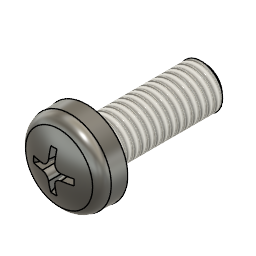
Assembly (Autodesk Fusion 360 archive; units mm, degrees)
design "Tornillo de cabeza plana redondeada ISO 7045 - M3 x 8 - H Acero 4.6 Normal"
description: Tornillo de cabeza plana redondeada ISO 7045 - M3 x 8 - H
part number: ISO 7045 - M3 x 8 - H Acero 4.6 Normal
Autodesk Fusion 360 part; units mm, degrees
sketch "Sketch1" plane through (0, 0, 0) normal (0, 1, 0) x (1, 0, 0)
  line L0 (-1.5, 1) -> (-1.5, 8)
  line L1 (-1.5, 8) -> (0, 8)
  line L2 (0, 8) -> (0, -2.4)
  line L3 (-1.3647, 0) -> (-2.8, 0)
  arc A0 (-2.7449, -1.5792) -> (0, -2.4) centre (0, 2.6) ccw
  line L4 (-1.5, 1) -> (-1.3647, 0.7098)
  line L5 (-1.3647, 0.7098) -> (-1.3647, 0)
  line L6 (-2.8, 0) -> (-2.7449, -1.5792)
  dimension "d9" = 3
  dimension "d66" = 5.6
  dimension "d75" = 2.7294
  dimension "d77" = 1
  dimension "d78" = 155
  dimension "d103" = 2
  dimension "d111" = 2.4
  dimension "d112" = 8
  constraint perpendicular L0 L1
  constraint collinear origin L2.end L1.end
  constraint perpendicular L0 L3
  constraint coincident origin L3
  constraint vertical L0
  constraint vertical L2
  constraint coincident L2 A0.centre
  constraint perpendicular L3 L5
  constraint coincident L3.start L5.end
  measures "d77" distance of L3 L0.start
  measures "d78" angle of L0 L4
  measures "d103" angle of L2 L6
  measures "d111" distance of L2.end L3
  measures "d112" distance of origin L1
revolve "Revolve1" add sketch "Sketch1" angle 360 about axis through (0, 0, -8) along (0, 0, 1) makes body 1
ref_plane "WorkPlane1" through (0, 0, 2.4) normal (0, 0, 1) x (1, 0, 0)
sketch "Sketch2" plane through (0, 0, 2.4) normal (0, 0, 1) x (1, 0, 0)
  line L0 (-0.215, 0.215) -> (-1.5, 0.215)
  line L1 (-0.215, -0.215) -> (-1.5, -0.215)
  line L2 (-1.5, 0.215) -> (-1.5, -0.215)
  line L3 (-0.215, -0.215) -> (-0.215, -1.5)
  line L4 (-0.215, -1.5) -> (0.215, -1.5)
  line L5 (0.215, -0.215) -> (0.215, -1.5)
  line L6 (0.215, -0.215) -> (1.5, -0.215)
  line L7 (1.5, -0.215) -> (1.5, 0.215)
  line L8 (0.215, 0.215) -> (1.5, 0.215)
  line L9 (0.215, 0.215) -> (0.215, 1.5)
  line L10 (0.215, 1.5) -> (-0.215, 1.5)
  line L11 (-0.215, 0.215) -> (-0.215, 1.5)
  dimension "d105" = 0.43
  dimension "d107" = 360
  dimension "d108" = 3
  constraint perpendicular L1 L2
  constraint vertical L0.start L1.start
  constraint horizontal L1
  constraint coincident L8.start L9.start
  measures "d105" distance of L0 L1
  measures "d108" distance of L2 L7
extrude "Extrude1" add sketch "Sketch2" against normal blind 1.8 draft -4 separate body makes body 2
draft "Draft1" angle -30 neutral plane through (0, 0, 2.4) pull (0, 0, 1) 4 faces at (-1.458, -0.0297, 1.8) (0.0297, -1.458, 1.8) (1.458, -0.0297, 1.8) (0.0297, 1.458, 1.8) on bodies 2
fillet "Fillet3" radius 0.43 4 edges at (0.1521, 0.1521, 1.5) (-0.1521, 0.1521, 1.5) (0.1521, -0.1521, 1.5) (-0.1521, -0.1521, 1.5) on bodies 2
combine "Combine1" operation cut target body 1 tool bodies 2
fillet "Fillet4" radius 0.9 1 edges at (-2.5591, 0.9926, 1.5792) on bodies 1
thread "Thread1" "ISO Metric profile 3.0 M3x0.5 M3x0.5 6g" major diameter 2.927 minor diameter 2.3555 pitch 0.5 angle 60 resizes the face on face at (-1.4925, 0.1494, -3.3333) on bodies 1
fillet "Fillet5" radius 0.3 1 edges at (-1.2723, 0.4935, 0) on bodies 1
sketch "Sketch5" plane through (0, 0, 0) normal (0, 1, 0) x (1, 0, 0)
  line L0 (-1.53, 8) -> (-1.53, 7.6933)
  line L1 (-1.53, 7.6933) -> (-1.1933, 8)
  line L2 (0, 8) -> (0, -2.4)
  line L3 (-1.53, 8) -> (0, 8)
  dimension "d114" = 0.3067
  dimension "d115" = 1.53
  dimension "d116" = 0.3367
  constraint coincident L2.start L3.end
  constraint perpendicular L2 L3
  constraint coincident L1.end L3
  constraint perpendicular L0 L3
  measures "d114" distance of L0.end L3
  measures "d115" distance of L0 L2.start
  measures "d116" distance of L0 L1.end
revolve "Revolve2" cut sketch "Sketch5" angle 360 about axis through (0, 0, -8) along (0, 0, 1) bodies 1
equation "d9 = adsk_nomdia"
equation "adsk_nomlen = 8.00 mm"
equation "adsk_headh = 2.40 mm"
equation "adsk_headdia = 5.60 mm"
equation "adsk_nomdia = 3.00 mm"
equation "adsk_phildia = 3.00 mm"
equation "d31 = -adsk_phildepth"
equation "adsk_philwidth = 0.43 mm"
equation "adsk_phildepth = 1.80 mm"
equation "d66 = adsk_headdia"
equation "d71 = adsk_headh"
equation "adsk_thrlen = 7.00 mm"
equation "d75 = adsk_shnkdia"
equation "adsk_shnkdia = 2.72937 mm"
equation "d77 = adsk_nomlen - adsk_thrlen"
equation "adsk_endpointdia = 2.38655 mm"
equation "adsk_startlen = 0.306725 mm"
equation "adsk_ovalrad = 5.00 mm"
equation "adsk_headtoprad = adsk_nomdia * 0.3"
equation "adsk_midfillet = adsk_nomdia * 0.1"
equation "d98 = adsk_midfillet"
equation "adsk_headang = 2.00 deg"
equation "d102 = adsk_headtoprad"
equation "d103 = adsk_headang"
equation "d105 = adsk_philwidth"
equation "d108 = adsk_phildia"
equation "d110 = adsk_philwidth"
equation "d111 = adsk_headh"
equation "d112 = adsk_nomlen"
equation "d113 = ( adsk_nomlen + adsk_headh ) - ( adsk_ovalrad )"
equation "d114 = adsk_startlen"
equation "d115 = adsk_nomdia * 0.51"
equation "d116 = ( adsk_nomdia * 0.51 ) - ( adsk_endpointdia / 2 )"

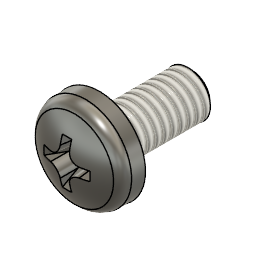
design "Tornillo de cabeza plana redondeada ISO 7045 - M4 x 8 - H Acero 4.6 Normal"
description: Tornillo de cabeza plana redondeada ISO 7045 - M4 x 8 - H
part number: ISO 7045 - M4 x 8 - H Acero 4.6 Normal
Autodesk Fusion 360 part; units mm, degrees
sketch "Sketch1" plane through (0, 0, 0) normal (0, 1, 0) x (1, 0, 0)
  line L0 (-2, 1.4) -> (-2, 8)
  line L1 (-2, 8) -> (0, 8)
  line L2 (0, 8) -> (0, -3.1)
  line L3 (-1.8106, 0) -> (-4, 0)
  arc A0 (-3.9381, -1.7712) -> (0, -3.1) centre (0, 3.4) ccw
  line L4 (-2, 1.4) -> (-1.8106, 0.9937)
  line L5 (-1.8106, 0.9937) -> (-1.8106, 0)
  line L6 (-4, 0) -> (-3.9381, -1.7712)
  dimension "d9" = 4
  dimension "d66" = 8
  dimension "d75" = 3.6211
  dimension "d77" = 1.4
  dimension "d78" = 155
  dimension "d103" = 2
  dimension "d111" = 3.1
  dimension "d112" = 8
  constraint perpendicular L0 L1
  constraint collinear origin L2.end L1.end
  constraint perpendicular L0 L3
  constraint coincident origin L3
  constraint vertical L0
  constraint vertical L2
  constraint coincident L2 A0.centre
  constraint perpendicular L3 L5
  constraint coincident L3.start L5.end
  measures "d77" distance of L3 L0.start
  measures "d78" angle of L0 L4
  measures "d103" angle of L2 L6
  measures "d111" distance of L2.end L3
  measures "d112" distance of origin L1
revolve "Revolve1" add sketch "Sketch1" angle 360 about axis through (0, 0, -8) along (0, 0, 1) makes body 1
ref_plane "WorkPlane1" through (0, 0, 3.1) normal (0, 0, 1) x (1, 0, 0)
sketch "Sketch2" plane through (0, 0, 3.1) normal (0, 0, 1) x (1, 0, 0)
  line L0 (-0.415, 0.415) -> (-2.2, 0.415)
  line L1 (-0.415, -0.415) -> (-2.2, -0.415)
  line L2 (-2.2, 0.415) -> (-2.2, -0.415)
  line L3 (-0.415, -0.415) -> (-0.415, -2.2)
  line L4 (-0.415, -2.2) -> (0.415, -2.2)
  line L5 (0.415, -0.415) -> (0.415, -2.2)
  line L6 (0.415, -0.415) -> (2.2, -0.415)
  line L7 (2.2, -0.415) -> (2.2, 0.415)
  line L8 (0.415, 0.415) -> (2.2, 0.415)
  line L9 (0.415, 0.415) -> (0.415, 2.2)
  line L10 (0.415, 2.2) -> (-0.415, 2.2)
  line L11 (-0.415, 0.415) -> (-0.415, 2.2)
  dimension "d105" = 0.83
  dimension "d107" = 360
  dimension "d108" = 4.4
  constraint perpendicular L1 L2
  constraint vertical L0.start L1.start
  constraint horizontal L1
  constraint coincident L8.start L9.start
  measures "d105" distance of L0 L1
  measures "d108" distance of L2 L7
extrude "Extrude1" add sketch "Sketch2" against normal blind 2.4 draft -4 separate body makes body 2
draft "Draft1" angle -30 neutral plane through (0, 0, 3.1) pull (0, 0, 1) 4 faces at (-2.1441, -0.0824, 2.3) (-0.0824, -2.1441, 2.3) (2.1441, 0.0824, 2.3) (-0.0824, 2.1441, 2.3) on bodies 2
fillet "Fillet3" radius 0.83 4 edges at (0.3311, 0.3311, 1.9) (-0.3311, 0.3311, 1.9) (0.3311, -0.3311, 1.9) (-0.3311, -0.3311, 1.9) on bodies 2
combine "Combine1" operation cut target body 1 tool bodies 2
fillet "Fillet4" radius 1.2 1 edges at (-3.6716, 1.4241, 1.7712) on bodies 1
thread "Thread1" "ISO Metric profile 4.0 M4x0.7 M4x0.7 6g" major diameter 3.908 minor diameter 3.111 pitch 0.7 angle 60 resizes the face on face at (-1.9901, 0.1991, -3.6) on bodies 1
fillet "Fillet5" radius 0.4 1 edges at (-1.688, 0.6547, 0) on bodies 1
sketch "Sketch5" plane through (0, 0, 0) normal (0, 1, 0) x (1, 0, 0)
  line L0 (-2.04, 8) -> (-2.04, 7.5706)
  line L1 (-2.04, 7.5706) -> (-1.5706, 8)
  line L2 (0, 8) -> (0, -3.1)
  line L3 (-2.04, 8) -> (0, 8)
  dimension "d114" = 0.4294
  dimension "d115" = 2.04
  dimension "d116" = 0.4694
  constraint coincident L2.start L3.end
  constraint perpendicular L2 L3
  constraint coincident L1.end L3
  constraint perpendicular L0 L3
  measures "d114" distance of L0.end L3
  measures "d115" distance of L0 L2.start
  measures "d116" distance of L0 L1.end
revolve "Revolve2" cut sketch "Sketch5" angle 360 about axis through (0, 0, -8) along (0, 0, 1) bodies 1
equation "d9 = adsk_nomdia"
equation "adsk_nomlen = 8.00 mm"
equation "adsk_headh = 3.10 mm"
equation "adsk_headdia = 8.00 mm"
equation "adsk_nomdia = 4.00 mm"
equation "adsk_phildia = 4.40 mm"
equation "d31 = -adsk_phildepth"
equation "adsk_philwidth = 0.83 mm"
equation "adsk_phildepth = 2.40 mm"
equation "d66 = adsk_headdia"
equation "d71 = adsk_headh"
equation "adsk_thrlen = 6.60 mm"
equation "d75 = adsk_shnkdia"
equation "adsk_shnkdia = 3.62111 mm"
equation "d77 = adsk_nomlen - adsk_thrlen"
equation "adsk_endpointdia = 3.14117 mm"
equation "adsk_startlen = 0.429415 mm"
equation "adsk_ovalrad = 6.50 mm"
equation "adsk_headtoprad = adsk_nomdia * 0.3"
equation "adsk_midfillet = adsk_nomdia * 0.1"
equation "d98 = adsk_midfillet"
equation "adsk_headang = 2.00 deg"
equation "d102 = adsk_headtoprad"
equation "d103 = adsk_headang"
equation "d105 = adsk_philwidth"
equation "d108 = adsk_phildia"
equation "d110 = adsk_philwidth"
equation "d111 = adsk_headh"
equation "d112 = adsk_nomlen"
equation "d113 = ( adsk_nomlen + adsk_headh ) - ( adsk_ovalrad )"
equation "d114 = adsk_startlen"
equation "d115 = adsk_nomdia * 0.51"
equation "d116 = ( adsk_nomdia * 0.51 ) - ( adsk_endpointdia / 2 )"
